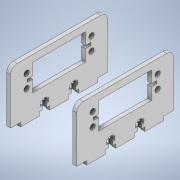
# Autodesk Inventor part: BaseMotoresHombrp
Saved by Autodesk Inventor 2022 (Build 260153000, 153)
## iProperties
Created: 2021-09-09
Part Number: BaseMotoresHombrp
Material: Generic
Document SubType Name: Modeling
Designer: Administrador
Density: 1 g/cm^3
Appearance: Default
Author: Administrador
Autodesk Inventor part; units mm, degrees
ref_plane "YZ Plane" through (0, 0, 0) normal (1, 0, 0) x (0, 1, 0)
ref_plane "XZ Plane" through (0, 0, 0) normal (0, 1, 0) x (-1, 0, 0)
ref_plane "XY Plane" through (0, 0, 0) normal (0, 0, 1) x (1, 0, 0)
sketch "Sketch1" plane through (0, 0, 0) normal (0, 0, 1) x (1, 0, 0)
  line L0 (0, 0) -> (3, 0)
  line L1 (3, 0) -> (3, 39.8)
  line L2 (3, 39.8) -> (0, 39.8)
  line L3 (0, 39.8) -> (0, 0)
  line L4 (-50.3, 0) -> (-47, 0) construction
  line L5 (-47, 0) -> (-47, 3.3) construction
  line L6 (-50.3, 3.3) -> (-47, 3.3) construction
  line L7 (-50.3, 0) -> (-50.3, 3.3) construction
  line L8 (0.2, 0) -> (3.3, 0)
  line L9 (0.2, 0) -> (3.3, 0)
  line L10 (-46.9, 0) -> (-49.9, 0)
  line L11 (-49.9, 0) -> (-49.9, 39.8)
  line L12 (-49.9, 39.8) -> (-46.9, 39.8)
  line L13 (-46.9, 39.8) -> (-46.9, 0)
  dimension "d0" = 3
  dimension "d1" = 39.8
  dimension "d22" = 3
  dimension "d23" = 46.9
  dimension "d150" = 39.8
  constraints: 20 end point, 4 horizontal, 4 parallel, 2 perpendicular, 2 other
  measures "d0" distance of L2.end L1.end
  measures "d1" distance of L1.end L0.end
  measures "d22" distance of L11.end L12.end
  measures "d23" distance between parallel lines of L13 L3
  measures "d150" distance of L12.end L10.start
extrude "Extrusion1" add sketch "Sketch1" along normal blind 73
sketch "Sketch2" plane through (0, 0, 0) normal (-1, 0, 0) x (0, 0, 1)
  line L0 (0, 0) -> (35, 0)
  line L1 (35, 0) -> (35, 14.8)
  line L2 (16.5, 14.8) -> (56.5, 14.8)
  line L3 (56.5, 34.8) -> (16.5, 34.8)
  line L4 (0, 39.8) -> (0, 0) projected
  line L5 (73, 39.8) -> (73, 0) projected
  line L6 (56.5, 14.8) -> (56.5, 23.8)
  line L7 (56.5, 23.8) -> (60.5, 23.8)
  line L8 (60.5, 23.8) -> (60.5, 25.8)
  line L9 (60.5, 25.8) -> (56.5, 25.8)
  line L10 (56.5, 14.8) -> (56.5, 23.8)
  line L11 (56.5, 25.8) -> (56.5, 34.8)
  line L12 (16.5, 14.8) -> (16.5, 23.8)
  line L13 (16.5, 23.8) -> (12.5, 23.8)
  line L14 (12.5, 23.8) -> (12.5, 25.8)
  line L15 (12.5, 25.8) -> (16.5, 25.8)
  line L16 (16.5, 34.8) -> (16.5, 25.8)
  line L17 (16.5, 23.8) -> (16.5, 14.8)
  dimension "d5" = 35
  dimension "d6" = 14.8
  dimension "d7" = 40
  dimension "d8" = 20
  dimension "d9" = 14.8
  dimension "d19" = 38
  dimension "d142" = 9
  dimension "d143" = 4
  dimension "d144" = 2
  dimension "d145" = 9
  dimension "d146" = 4
  constraints: 32 end point, 10 perpendicular, 5 parallel, 3 horizontal
  measures "d5" distance of L0.start L0.end
  measures "d6" distance of L0.end L1.end
  measures "d7" distance of L3.end L3.start
  measures "d8" distance of L3.start L2.end
  measures "d9" distance between parallel lines of L0 L2
  measures "d19" distance between parallel lines of L5 L1
  measures "d142" distance of L2.end L6.end
  measures "d143" distance of L6.end L7.end
  measures "d144" distance of L7.end L8.end
  measures "d145" distance of L2.start L12.end
  measures "d146" distance of L12.end L13.end
extrude "Extrusion2" cut sketch "Sketch2" against normal blind 3 and the other way blind 8.05
fillet "Fillet1" radius 5 4 edges at (1.5, 39.8, 0) (1.5, 39.8, 73) (-48.4, 39.8, 0) (-48.4, 39.8, 73)
sketch "Sketch4" plane through (-49.9, 0, 0) normal (-1, 0, 0) x (0, 0, 1)
  line L0 (56.5, 14.8) -> (16.5, 14.8) projected
  line L1 (16.5, 25.8) -> (16.5, 34.8) projected
  line L2 (16.5, 34.8) -> (56.5, 34.8) projected
  line L3 (16.5, 34.8) -> (56.5, 34.8)
  line L4 (56.5, 14.8) -> (16.5, 14.8)
  line L5 (16.5, 23.8) -> (12.5, 23.8) projected
  line L6 (12.5, 25.8) -> (16.5, 25.8) projected
  line L7 (12.5, 23.8) -> (12.5, 25.8) projected
  line L8 (60.5, 23.8) -> (56.5, 23.8) projected
  line L9 (56.5, 25.8) -> (60.5, 25.8) projected
  line L10 (60.5, 25.8) -> (60.5, 23.8) projected
  line L11 (16.5, 23.8) -> (12.5, 23.8)
  line L12 (12.5, 23.8) -> (12.5, 25.8)
  line L13 (16.5, 25.8) -> (12.5, 25.8)
  line L14 (56.5, 23.8) -> (60.5, 23.8)
  line L15 (60.5, 23.8) -> (60.5, 25.8)
  line L16 (60.5, 25.8) -> (56.5, 25.8)
  line L17 (56.5, 34.8) -> (56.5, 25.8)
  line L18 (56.5, 23.8) -> (56.5, 14.8)
  line L19 (16.5, 14.8) -> (16.5, 23.8)
  line L20 (16.5, 25.8) -> (16.5, 34.8)
  point P0 (0, 0)
  point P1 (56.5, 34.8)
  constraints: 24 end point, 9 equal length, 3 perpendicular, 2 horizontal
extrude "Extrusion4" cut sketch "Sketch4" against normal blind 3
sketch "Sketch6" plane through (3, 0, 73) normal (1, 0, 0) x (0, 0, -1)
  line L0 (65.5, 0) -> (65.5, -3)
  line L1 (65.5, -3) -> (51.5, -3)
  line L2 (51.5, -3) -> (51.5, 0)
  line L3 (43.5, 0) -> (43.5, -3)
  line L4 (43.5, -3) -> (29.5, -3)
  line L5 (29.5, -3) -> (29.5, 0)
  line L6 (21.5, 0) -> (21.5, -3)
  line L7 (21.5, -3) -> (7.5, -3)
  line L8 (7.5, -3) -> (7.5, 0)
  line L9 (21.5, 0) -> (7.5, 0)
  line L10 (65.5, 0) -> (51.5, 0)
  line L11 (43.5, 0) -> (29.5, 0)
  line L12 (0, 0) -> (0, 34.8) projected
  line L13 (73, 0) -> (73, 34.8) projected
  dimension "d78" = 3
  dimension "d79" = 14
  dimension "d80" = 8
  dimension "d81" = 14
  dimension "d82" = 8
  dimension "d83" = 14
  dimension "d84" = 7.5
  dimension "d85" = 7.5
  constraints: 24 end point, 5 perpendicular, 2 point on line, 1 vertical
  measures "d78" distance of L0.start L0.end
  measures "d79" distance of L0.end L1.end
  measures "d80" distance of L2.end L3.start
  measures "d81" distance of L3.end L4.end
  measures "d82" distance of L5.end L6.start
  measures "d83" distance of L6.end L7.end
  measures "d84" distance between parallel lines of L8 L12
  measures "d85" distance between parallel lines of L13 L0
extrude "Extrusion5" add sketch "Sketch6" against normal blind 3
sketch "Sketch7" plane through (3, 0, 0) normal (1, 0, 0) x (0, 0, -1)
  line L0 (0, 0) -> (0, 34.8) projected
  line L1 (-49.05, 0) -> (-49.05, 3)
  line L2 (-49.05, 3) -> (-50.55, 3)
  line L3 (-50.55, 3) -> (-50.55, 6)
  line L4 (-50.55, 6) -> (-49.05, 6)
  line L5 (-49.05, 6) -> (-49.05, 7)
  line L6 (-49.05, 7) -> (-45.95, 7)
  line L7 (-45.95, 7) -> (-45.95, 6)
  line L8 (-45.95, 6) -> (-44.45, 6)
  line L9 (-44.45, 3) -> (-45.95, 3)
  line L10 (-45.95, 3) -> (-45.95, 0)
  line L11 (-44.45, 6) -> (-44.45, 3)
  line L12 (-49.05, 0) -> (-45.95, 0)
  line L13 (-51.5, -3) -> (-51.5, 0) projected
  line L14 (-21.5, 0) -> (-29.5, 0) projected
  line L15 (-29.5, 0) -> (-27.05, 0)
  line L16 (-27.05, 0) -> (-23.95, 0)
  line L17 (-27.05, 0) -> (-27.05, 3)
  line L18 (-27.05, 3) -> (-28.55, 3)
  line L19 (-28.55, 3) -> (-28.55, 6)
  line L20 (-28.55, 6) -> (-27.05, 6)
  line L21 (-27.05, 6) -> (-27.05, 7)
  line L22 (-27.05, 7) -> (-23.95, 7)
  line L23 (-23.95, 7) -> (-23.95, 6)
  line L24 (-23.95, 6) -> (-22.45, 6)
  line L25 (-22.45, 6) -> (-22.45, 3)
  line L26 (-22.45, 3) -> (-23.95, 3)
  line L27 (-23.95, 3) -> (-23.95, 0)
  line L28 (-43.5, -3) -> (-29.5, -3) projected
  dimension "d89" = 3
  dimension "d92" = 3.1
  dimension "d96" = 1.5
  dimension "d98" = 2.45
  dimension "d99" = 2.45
  dimension "d100" = 3.1
  dimension "d101" = 3
  dimension "d102" = 1.5
  dimension "d104" = 1.5
  dimension "d107" = 1.5
  dimension "d108" = 1
  dimension "d109" = 3.1
  dimension "d110" = 1
  dimension "d111" = 3
  dimension "d112" = 3
  dimension "d113" = 6.1
  dimension "d114" = 6.1
  dimension "d116" = 3
  dimension "d117" = 3
  dimension "d118" = 10
  dimension "d119" = 3
  constraints: 50 end point, 12 perpendicular, 9 point on line, 4 vertical, 1 horizontal
  measures "d89" distance of L1.start L1.end
  measures "d92" distance of L5.end L6.end
  measures "d96" distance of L9.start L9.end
  measures "d98" distance from line of L1.start L13
  measures "d99" distance of L14.end L15.end
  measures "d100" distance of L15.end L16.end
  measures "d101" distance of L15.end L17.end
  measures "d102" distance of L17.end L18.end
  measures "d104" distance of L19.end L20.end
  measures "d107" distance of L23.end L24.end
  measures "d108" distance from line of L22 L19.end
  measures "d109" distance of L21.end L22.end
  measures "d110" distance of L22.end L23.end
  measures "d111" distance of L24.end L25.end
  measures "d112" distance of L26.end L16.end
  measures "d113" distance between parallel lines of L11 L3
  measures "d114" distance between parallel lines of L25 L19
  measures "d116" distance between parallel lines of L2 L4
  measures "d117" distance of L8.end L9.start
  measures "d118" distance between parallel lines of L6 L28
  measures "d119" distance between parallel lines of L14 L26
extrude "Extrusion6" cut sketch "Sketch7" against normal blind 3
sketch "Sketch8" plane through (-49.9, 0, 0) normal (-1, 0, 0) x (0, 0, 1)
  circle A0 centre (61, 29.8) radius 2
  circle A1 centre (12, 29.8) radius 2
  circle A2 centre (12, 19.8) radius 2
  circle A3 centre (61, 19.8) radius 2
  line L0 (16.5, 34.8) -> (56.5, 34.8) projected
  line L1 (56.5, 14.8) -> (16.5, 14.8) projected
  point P0 (0, 0)
  dimension "d127" = 4
  dimension "d128" = 4
  dimension "d130" = 4
  dimension "d131" = 4
  dimension "d134" = 5
  dimension "d135" = 5
  dimension "d136" = 10
  dimension "d137" = 10
  dimension "d138" = 5
  dimension "d139" = 5
  dimension "d140" = 49
  dimension "d141" = 49
  constraints: 4 centre point
  measures "d127" diameter of A0
  measures "d128" diameter of A1
  measures "d130" diameter of A2
  measures "d131" diameter of A3
  measures "d134" distance from line of A0.centre L0
  measures "d135" distance from line of L1 A3.centre
  measures "d136" distance of A0.centre A3.centre
  measures "d137" distance of A1.centre A2.centre
  measures "d138" distance from line of A2.centre L1
  measures "d139" distance from line of A1.centre L0
  measures "d140" distance of A3.centre A2.centre
  measures "d141" distance of A1.centre A0.centre
extrude "Extrusion7" cut sketch "Sketch8" against normal up to surface (3 mm away)
sketch "Sketch9" plane through (3, 0, 0) normal (1, 0, 0) x (0, 0, -1)
  circle A0 centre (-12, 29.8) radius 2 projected
  circle A1 centre (-12, 19.8) radius 2 projected
  circle A2 centre (-61, 29.8) radius 2 projected
  circle A3 centre (-61, 19.8) radius 2 projected
  circle A4 centre (-61, 29.8) radius 2
  circle A5 centre (-61, 19.8) radius 2
  circle A6 centre (-12, 19.8) radius 2
  circle A7 centre (-12, 29.8) radius 2
  point P0 (0, 0)
  constraints: 4 centre point, 4 coincident, 4 concentric
extrude "Extrusion8" cut sketch "Sketch9" against normal up to surface (3 mm away)
sketch "Sketch10" plane through (-46.9, 0, 73) normal (1, 0, 0) x (0, 0, -1)
  line L0 (7.5, -3) -> (21.5, -3) projected
  line L1 (73, 0) -> (0, 0) projected
  line L2 (7.5, -3) -> (21.5, -3)
  line L3 (21.5, -3) -> (21.5, 0)
  line L4 (21.5, 0) -> (7.5, 0)
  line L5 (7.5, 0) -> (7.5, -3)
  line L6 (43.5, -3) -> (29.5, -3) projected
  line L7 (29.5, -3) -> (43.5, -3)
  line L8 (43.5, -3) -> (43.5, 0)
  line L9 (43.5, 0) -> (29.5, 0)
  line L10 (29.5, 0) -> (29.5, -3)
  line L11 (65.5, -3) -> (51.5, -3) projected
  line L12 (51.5, -3) -> (65.5, -3)
  line L13 (65.5, -3) -> (65.5, 0)
  line L14 (65.5, 0) -> (51.5, 0)
  line L15 (51.5, 0) -> (51.5, -3)
  point P0 (51.5, 0)
  point P1 (65.5, -3)
  point P2 (65.5, 0)
  point P3 (29.5, 0)
  point P4 (43.5, -3)
  point P5 (43.5, 0)
  point P6 (7.5, 0)
  point P7 (21.5, -3)
  dimension "d147" = 14
  dimension "d148" = 14
  dimension "d149" = 14
  constraints: 24 end point, 6 parallel, 3 horizontal, 3 perpendicular, 3 point on line
  measures "d147" distance of L4.end L3.end
  measures "d148" distance of L9.end L8.end
  measures "d149" distance of L14.end L13.end
extrude "Extrusion9" add sketch "Sketch10" against normal blind 3
sketch "Sketch11" plane through (-46.9, 0, 0) normal (1, 0, 0) x (0, 0, -1)
  line L0 (0, 0) -> (0, 34.8)
  arc A0 (-5, 39.8) -> (0, 34.8) centre (-5, 34.8) ccw projected
  line L1 (-23.95, 3) -> (-23.95, 0) projected
  line L2 (-49.05, 0) -> (-49.05, 3) projected
  line L3 (-49.05, 3) -> (-50.55, 3) projected
  line L4 (-50.55, 3) -> (-50.55, 6) projected
  line L5 (-50.55, 6) -> (-49.05, 6) projected
  line L6 (-49.05, 6) -> (-49.05, 7) projected
  line L7 (-49.05, 7) -> (-45.95, 7) projected
  line L8 (-45.95, 7) -> (-45.95, 6) projected
  line L9 (-27.05, 0) -> (-27.05, 3) projected
  line L10 (-27.05, 3) -> (-28.55, 3) projected
  line L11 (-28.55, 3) -> (-28.55, 6) projected
  line L12 (-49.05, 0) -> (-49.05, 3)
  line L13 (-50.55, 3) -> (-49.05, 3)
  line L14 (-50.55, 3) -> (-50.55, 6)
  line L15 (-50.55, 6) -> (-49.05, 6)
  line L16 (-49.05, 6) -> (-49.05, 7)
  line L17 (-49.05, 7) -> (-45.95, 7)
  line L18 (-45.95, 7) -> (-45.95, 6)
  line L19 (-28.55, 3) -> (-28.55, 6)
  line L20 (-27.05, 3) -> (-27.05, 0)
  line L21 (-23.95, 0) -> (-23.95, 3)
  line L22 (-27.05, 3) -> (-28.55, 3)
  line L23 (-23.95, 6) -> (-22.45, 6)
  line L24 (-27.05, 7) -> (-23.95, 7)
  line L25 (-23.95, 7) -> (-23.95, 6)
  line L26 (-22.45, 6) -> (-22.45, 3)
  line L27 (-22.45, 3) -> (-23.95, 3)
  line L28 (-27.05, 0) -> (-23.95, 0)
  line L29 (-21.5, 0) -> (-29.5, 0) projected
  line L30 (-27.05, 7) -> (-27.05, 6)
  line L31 (-27.05, 6) -> (-28.55, 6)
  line L32 (-45.95, 6) -> (-44.45, 6)
  line L33 (-44.45, 6) -> (-44.45, 3)
  line L34 (-44.45, 3) -> (-45.95, 3)
  line L35 (-45.95, 3) -> (-45.95, 0)
  line L36 (-45.95, 0) -> (-49.05, 0)
  point P0 (-23.95, 3)
  point P1 (-23.95, 0)
  constraints: 50 end point, 9 perpendicular, 4 collinear, 3 horizontal, 2 vertical, 1 centre point, 1 parallel
extrude "Extrusion10" cut sketch "Sketch11" against normal blind 3
body "Solid1"
